Autodesk Inventor part; units mm, degrees
(part 2 of 3)
sketch "Эскиз4" plane through (0, 2, 0) normal (0, 1, 0) x (1, 0, 0)
  arc A0 (37.7453, 90.4395) -> (18.0526, 96.3229) centre (0, 0) ccw projected
  arc A1 (38.3892, 87.1795) -> (37.7453, 90.4395) centre (36.975, 88.5938) ccw projected
  line L0 (38.3892, 87.1795) -> (34.2947, 83.085) projected
  arc A2 (34.2947, 83.085) -> (34.2947, 76.014) centre (37.8302, 79.5495) ccw projected
  line L1 (34.2947, 76.014) -> (42.4264, 67.8823) projected
  line L2 (42.4264, 67.8823) -> (21.6698, 47.1257) projected
  arc A3 (21.6698, 47.1257) -> (17.9282, 43.384) centre (21.9203, 43.1335) ccw projected
  line L3 (17.9282, 43.384) -> (1.4142, 26.8701) projected
  arc A4 (-1.4142, 26.8701) -> (1.4142, 26.8701) centre (0, 28.2843) ccw projected
  line L4 (-1.4142, 26.8701) -> (-17.9282, 43.384) projected
  arc A5 (-17.9282, 43.384) -> (-21.6698, 47.1257) centre (-21.9203, 43.1335) ccw projected
  line L5 (-21.6698, 47.1257) -> (-42.4264, 67.8823) projected
  line L6 (-42.4264, 67.8823) -> (-34.2947, 76.014) projected
  arc A6 (-34.2947, 76.014) -> (-34.2947, 83.085) centre (-37.8302, 79.5495) ccw projected
  line L7 (-34.2947, 83.085) -> (-38.3892, 87.1795) projected
  arc A7 (-37.7453, 90.4395) -> (-38.3892, 87.1795) centre (-36.975, 88.5938) ccw projected
  arc A8 (-18.0526, 96.3229) -> (-37.7453, 90.4395) centre (0, 0) ccw projected
  arc A9 (-14.5, 93.3742) -> (-18.0526, 96.3229) centre (-17.5, 93.3742) ccw projected
  line L8 (-14.5, 93.3742) -> (-14.5, 87) projected
  arc A10 (-14.5, 87) -> (-11.5, 84) centre (-11.5, 87) ccw projected
  line L9 (-11.5, 84) -> (11.5, 84) projected
  arc A11 (11.5, 84) -> (14.5, 87) centre (11.5, 87) ccw projected
  line L10 (14.5, 87) -> (14.5, 93.3742) projected
  arc A12 (18.0526, 96.3229) -> (14.5, 93.3742) centre (17.5, 93.3742) ccw projected
  line L11 (8.5, 101.3496) -> (8.5, 90.5) projected
  arc A13 (7, 89) -> (8.5, 90.5) centre (7, 90.5) ccw projected
  line L12 (7, 89) -> (-7, 89) projected
  arc A14 (-8.5, 90.5) -> (-7, 89) centre (-7, 90.5) ccw projected
  line L13 (-8.5, 90.5) -> (-8.5, 101.3496) projected
  arc A15 (-8.5, 101.3496) -> (-11.8382, 104.3305) centre (-11.5, 101.3496) ccw projected
  arc A16 (-11.8382, 104.3305) -> (-48.6481, 93.0503) centre (0, 0) ccw projected
  arc A17 (-48.6481, 93.0503) -> (-49.3795, 88.2704) centre (-47.2582, 90.3917) ccw projected
  line L14 (-49.3795, 88.2704) -> (-46.3155, 85.2064) projected
  arc A18 (-46.3155, 73.8927) -> (-46.3155, 85.2064) centre (-51.9723, 79.5495) ccw projected
  line L15 (-46.3155, 73.8927) -> (-73.8927, 46.3155) projected
  arc A19 (-85.2064, 46.3155) -> (-73.8927, 46.3155) centre (-79.5495, 51.9723) ccw projected
  line L16 (-85.2064, 46.3155) -> (-88.2704, 49.3795) projected
  arc A20 (-88.2704, 49.3795) -> (-93.0503, 48.6481) centre (-90.3917, 47.2582) ccw projected
  arc A21 (-93.0503, 48.6481) -> (-93.0503, -48.6481) centre (0, 0) ccw projected
  arc A22 (-93.0503, -48.6481) -> (-88.2704, -49.3795) centre (-90.3917, -47.2582) ccw projected
  line L17 (-88.2704, -49.3795) -> (-85.2064, -46.3155) projected
  arc A23 (-73.8927, -46.3155) -> (-85.2064, -46.3155) centre (-79.5495, -51.9723) ccw projected
  line L18 (-73.8927, -46.3155) -> (-46.3155, -73.8927) projected
  arc A24 (-46.3155, -85.2064) -> (-46.3155, -73.8927) centre (-51.9723, -79.5495) ccw projected
  line L19 (-46.3155, -85.2064) -> (-49.3795, -88.2704) projected
  arc A25 (-49.3795, -88.2704) -> (-48.6481, -93.0503) centre (-47.2582, -90.3917) ccw projected
  arc A26 (-48.6481, -93.0503) -> (-45.42, -94.668) centre (0, 0) ccw projected
  arc A27 (-45.42, -94.668) -> (-43.0355, -94.1655) centre (-44.5548, -92.8648) ccw projected
  line L20 (-43.0355, -94.1655) -> (-18.3802, -65.3664) projected
  arc A28 (-17.477, -64.7643) -> (-18.3802, -65.3664) centre (-16.8609, -66.6671) ccw projected
  line L21 (-17.477, -64.7643) -> (-0.6161, -59.3045) projected
  arc A29 (0.6161, -59.3045) -> (-0.6161, -59.3045) centre (0, -61.2072) ccw projected
  line L22 (0.6161, -59.3045) -> (17.477, -64.7643) projected
  arc A30 (18.3802, -65.3664) -> (17.477, -64.7643) centre (16.8609, -66.6671) ccw projected
  line L23 (18.3802, -65.3664) -> (43.0355, -94.1655) projected
  arc A31 (43.0355, -94.1655) -> (45.42, -94.668) centre (44.5548, -92.8648) ccw projected
  arc A32 (45.42, -94.668) -> (48.6481, -93.0503) centre (0, 0) ccw projected
  arc A33 (48.6481, -93.0503) -> (49.3795, -88.2704) centre (47.2582, -90.3917) ccw projected
  line L24 (49.3795, -88.2704) -> (46.3155, -85.2064) projected
  arc A34 (46.3155, -73.8927) -> (46.3155, -85.2064) centre (51.9723, -79.5495) ccw projected
  line L25 (46.3155, -73.8927) -> (73.8927, -46.3155) projected
  arc A35 (85.2064, -46.3155) -> (73.8927, -46.3155) centre (79.5495, -51.9723) ccw projected
  line L26 (85.2064, -46.3155) -> (88.2704, -49.3795) projected
  arc A36 (88.2704, -49.3795) -> (93.0503, -48.6481) centre (90.3917, -47.2582) ccw projected
  arc A37 (93.0503, -48.6481) -> (93.0503, 48.6481) centre (0, 0) ccw projected
  arc A38 (93.0503, 48.6481) -> (88.2704, 49.3795) centre (90.3917, 47.2582) ccw projected
  line L27 (88.2704, 49.3795) -> (85.2064, 46.3155) projected
  arc A39 (73.8927, 46.3155) -> (85.2064, 46.3155) centre (79.5495, 51.9723) ccw projected
  line L28 (73.8927, 46.3155) -> (46.3155, 73.8927) projected
  arc A40 (46.3155, 85.2064) -> (46.3155, 73.8927) centre (51.9723, 79.5495) ccw projected
  line L29 (46.3155, 85.2064) -> (49.3795, 88.2704) projected
  arc A41 (49.3795, 88.2704) -> (48.6481, 93.0503) centre (47.2582, 90.3917) ccw projected
  arc A42 (48.6481, 93.0503) -> (11.8382, 104.3305) centre (0, 0) ccw projected
  arc A43 (11.8382, 104.3305) -> (8.5, 101.3496) centre (11.5, 101.3496) ccw projected
  line L30 (67.8823, -42.4264) -> (47.1257, -21.6698) projected
  arc A44 (47.1257, -21.6698) -> (43.384, -17.9282) centre (43.1335, -21.9203) ccw projected
  line L31 (43.384, -17.9282) -> (26.8701, -1.4142) projected
  arc A45 (26.8701, 1.4142) -> (26.8701, -1.4142) centre (28.2843, 0) ccw projected
  line L32 (26.8701, 1.4142) -> (43.384, 17.9282) projected
  arc A46 (43.384, 17.9282) -> (47.1257, 21.6698) centre (43.1335, 21.9203) ccw projected
  line L33 (47.1257, 21.6698) -> (67.8823, 42.4264) projected
  line L34 (67.8823, 42.4264) -> (76.014, 34.2947) projected
  arc A47 (76.014, 34.2947) -> (83.085, 34.2947) centre (79.5495, 37.8302) ccw projected
  line L35 (83.085, 34.2947) -> (87.1795, 38.3892) projected
  arc A48 (90.4395, 37.7453) -> (87.1795, 38.3892) centre (88.5938, 36.975) ccw projected
  arc A49 (90.4395, -37.7453) -> (90.4395, 37.7453) centre (0, 0) ccw projected
  arc A50 (87.1795, -38.3892) -> (90.4395, -37.7453) centre (88.5938, -36.975) ccw projected
  line L36 (87.1795, -38.3892) -> (83.085, -34.2947) projected
  arc A51 (83.085, -34.2947) -> (76.014, -34.2947) centre (79.5495, -37.8302) ccw projected
  line L37 (76.014, -34.2947) -> (67.8823, -42.4264) projected
  circle A52 centre (-37.8302, -79.5495) radius 1.6 projected
  circle A53 centre (37.8302, -79.5495) radius 1.6 projected
  circle A54 centre (20.5578, -60.8546) radius 1.55 projected
  circle A55 centre (-20.5578, -60.8546) radius 1.55 projected
  circle A56 centre (79.5495, 37.8302) radius 1.6 projected
  circle A57 centre (37.8302, 79.5495) radius 1.6 projected
  circle A58 centre (79.5495, -37.8302) radius 1.6 projected
  circle A59 centre (-79.5495, -37.8302) radius 1.6 projected
  circle A60 centre (-79.5495, 37.8302) radius 1.6 projected
  circle A61 centre (-37.8302, 79.5495) radius 1.6 projected
  circle A62 centre (22, 0) radius 1.6 projected
  circle A63 centre (0, -22) radius 1.6 projected
  circle A64 centre (-22, 0) radius 1.6 projected
  circle A65 centre (0, 22) radius 1.6 projected
  circle A66 centre (43.1335, -21.9203) radius 1.6 projected
  circle A67 centre (0, 0) radius 18 projected
  circle A68 centre (-43.1335, 21.9203) radius 1.6 projected
  circle A69 centre (-21.9203, -43.1335) radius 1.6 projected
  circle A70 centre (21.9203, 43.1335) radius 1.6 projected
  circle A71 centre (43.1335, 21.9203) radius 1.6 projected
  circle A72 centre (-43.1335, -21.9203) radius 1.6 projected
  arc A73 (-21.4111, -8.4003) -> (-8.4003, -21.4111) centre (0, 0) ccw projected
  arc A74 (-7.7166, -24.6871) -> (-8.4003, -21.4111) centre (-9.1308, -23.2729) ccw projected
  line L38 (-7.7166, -24.6871) -> (-20.8597, -37.8302) projected
  arc A75 (-23.6881, -37.8302) -> (-20.8597, -37.8302) centre (-22.2739, -36.416) ccw projected
  line L39 (-23.6881, -37.8302) -> (-37.8302, -23.6881) projected
  arc A76 (-37.8302, -20.8597) -> (-37.8302, -23.6881) centre (-36.416, -22.2739) ccw projected
  line L40 (-37.8302, -20.8597) -> (-24.6871, -7.7166) projected
  arc A77 (-21.4111, -8.4003) -> (-24.6871, -7.7166) centre (-23.2729, -9.1308) ccw projected
  circle A78 centre (21.9203, -43.1335) radius 1.6 projected
  line L41 (37.8302, 20.8597) -> (24.6871, 7.7166) projected
  arc A79 (21.4111, 8.4003) -> (24.6871, 7.7166) centre (23.2729, 9.1308) ccw projected
  arc A80 (21.4111, 8.4003) -> (8.4003, 21.4111) centre (0, 0) ccw projected
  arc A81 (7.7166, 24.6871) -> (8.4003, 21.4111) centre (9.1308, 23.2729) ccw projected
  line L42 (7.7166, 24.6871) -> (20.8597, 37.8302) projected
  arc A82 (23.6881, 37.8302) -> (20.8597, 37.8302) centre (22.2739, 36.416) ccw projected
  line L43 (23.6881, 37.8302) -> (37.8302, 23.6881) projected
  arc A83 (37.8302, 20.8597) -> (37.8302, 23.6881) centre (36.416, 22.2739) ccw projected
  arc A84 (-24.6871, 7.7166) -> (-21.4111, 8.4003) centre (-23.2729, 9.1308) ccw projected
  line L44 (-24.6871, 7.7166) -> (-37.8302, 20.8597) projected
  arc A85 (-37.8302, 23.6881) -> (-37.8302, 20.8597) centre (-36.416, 22.2739) ccw projected
  line L45 (-37.8302, 23.6881) -> (-23.6881, 37.8302) projected
  arc A86 (-20.8597, 37.8302) -> (-23.6881, 37.8302) centre (-22.2739, 36.416) ccw projected
  line L46 (-20.8597, 37.8302) -> (-7.7166, 24.6871) projected
  arc A87 (-8.4003, 21.4111) -> (-7.7166, 24.6871) centre (-9.1308, 23.2729) ccw projected
  arc A88 (-8.4003, 21.4111) -> (-21.4111, 8.4003) centre (0, 0) ccw projected
  circle A89 centre (-21.9203, 43.1335) radius 1.6 projected
  arc A90 (24.6871, -7.7166) -> (21.4111, -8.4003) centre (23.2729, -9.1308) ccw projected
  line L47 (24.6871, -7.7166) -> (37.8302, -20.8597) projected
  arc A91 (37.8302, -23.6881) -> (37.8302, -20.8597) centre (36.416, -22.2739) ccw projected
  line L48 (37.8302, -23.6881) -> (23.6881, -37.8302) projected
  arc A92 (20.8597, -37.8302) -> (23.6881, -37.8302) centre (22.2739, -36.416) ccw projected
  line L49 (20.8597, -37.8302) -> (7.7166, -24.6871) projected
  arc A93 (8.4003, -21.4111) -> (7.7166, -24.6871) centre (9.1308, -23.2729) ccw projected
  arc A94 (8.4003, -21.4111) -> (21.4111, -8.4003) centre (0, 0) ccw projected
  line L50 (46.669, -63.6396) -> (27.2236, -44.1942) projected
  arc A95 (27.2236, -41.3657) -> (27.2236, -44.1942) centre (28.6378, -42.78) ccw projected
  line L51 (27.2236, -41.3657) -> (41.3657, -27.2236) projected
  arc A96 (44.1942, -27.2236) -> (41.3657, -27.2236) centre (42.78, -28.6378) ccw projected
  line L52 (44.1942, -27.2236) -> (63.6396, -46.669) projected
  line L53 (63.6396, -46.669) -> (46.669, -63.6396) projected
  line L54 (-42.4264, -67.8823) -> (-21.6698, -47.1257) projected
  arc A97 (-21.6698, -47.1257) -> (-17.9282, -43.384) centre (-21.9203, -43.1335) ccw projected
  line L55 (-17.9282, -43.384) -> (-1.4142, -26.8701) projected
  arc A98 (1.4142, -26.8701) -> (-1.4142, -26.8701) centre (0, -28.2843) ccw projected
  line L56 (1.4142, -26.8701) -> (17.9282, -43.384) projected
  arc A99 (17.9282, -43.384) -> (21.6698, -47.1257) centre (21.9203, -43.1335) ccw projected
  line L57 (21.6698, -47.1257) -> (42.4264, -67.8823) projected
  line L58 (42.4264, -67.8823) -> (37.1244, -73.1843) projected
  arc A100 (34.1909, -73.0707) -> (37.1244, -73.1843) centre (35.7102, -71.7701) ccw projected
  line L59 (34.1909, -73.0707) -> (25.4187, -62.8242) projected
  arc A101 (24.842, -61.8893) -> (25.4187, -62.8242) centre (28.1154, -60.5155) ccw projected
  line L60 (24.842, -61.8893) -> (23.8313, -59.4808) projected
  arc A102 (23.8313, -59.4808) -> (21.0049, -57.3328) centre (20.5578, -60.8546) ccw projected
  line L61 (21.0049, -57.3328) -> (15.1585, -56.5907) projected
  arc A103 (14.5119, -56.4463) -> (15.1585, -56.5907) centre (15.6055, -53.069) ccw projected
  line L62 (14.5119, -56.4463) -> (0.6161, -51.9466) projected
  arc A104 (0.6161, -51.9466) -> (-0.6161, -51.9466) centre (0, -53.8493) ccw projected
  line L63 (-0.6161, -51.9466) -> (-14.5119, -56.4463) projected
  arc A105 (-15.1585, -56.5907) -> (-14.5119, -56.4463) centre (-15.6055, -53.069) ccw projected
  line L64 (-15.1585, -56.5907) -> (-21.0049, -57.3328) projected
  arc A106 (-21.0049, -57.3328) -> (-23.8313, -59.4808) centre (-20.5578, -60.8546) ccw projected
  line L65 (-23.8313, -59.4808) -> (-24.842, -61.8893) projected
  arc A107 (-25.4187, -62.8242) -> (-24.842, -61.8893) centre (-28.1154, -60.5155) ccw projected
  line L66 (-25.4187, -62.8242) -> (-34.1909, -73.0707) projected
  arc A108 (-37.1244, -73.1843) -> (-34.1909, -73.0707) centre (-35.7102, -71.7701) ccw projected
  line L67 (-37.1244, -73.1843) -> (-42.4264, -67.8823) projected
  line L68 (-63.6396, -46.669) -> (-44.1942, -27.2236) projected
  arc A109 (-41.3657, -27.2236) -> (-44.1942, -27.2236) centre (-42.78, -28.6378) ccw projected
  line L69 (-41.3657, -27.2236) -> (-27.2236, -41.3657) projected
  arc A110 (-27.2236, -44.1942) -> (-27.2236, -41.3657) centre (-28.6378, -42.78) ccw projected
  line L70 (-27.2236, -44.1942) -> (-46.669, -63.6396) projected
  line L71 (-46.669, -63.6396) -> (-63.6396, -46.669) projected
  line L72 (-67.8823, 42.4264) -> (-47.1257, 21.6698) projected
  arc A111 (-47.1257, 21.6698) -> (-43.384, 17.9282) centre (-43.1335, 21.9203) ccw projected
  line L73 (-43.384, 17.9282) -> (-26.8701, 1.4142) projected
  arc A112 (-26.8701, -1.4142) -> (-26.8701, 1.4142) centre (-28.2843, 0) ccw projected
  line L74 (-26.8701, -1.4142) -> (-43.384, -17.9282) projected
  arc A113 (-43.384, -17.9282) -> (-47.1257, -21.6698) centre (-43.1335, -21.9203) ccw projected
  line L75 (-47.1257, -21.6698) -> (-67.8823, -42.4264) projected
  line L76 (-67.8823, -42.4264) -> (-76.014, -34.2947) projected
  arc A114 (-76.014, -34.2947) -> (-83.085, -34.2947) centre (-79.5495, -37.8302) ccw projected
  line L77 (-83.085, -34.2947) -> (-87.1795, -38.3892) projected
  arc A115 (-90.4395, -37.7453) -> (-87.1795, -38.3892) centre (-88.5938, -36.975) ccw projected
  arc A116 (-90.4395, 37.7453) -> (-90.4395, -37.7453) centre (0, 0) ccw projected
  arc A117 (-87.1795, 38.3892) -> (-90.4395, 37.7453) centre (-88.5938, 36.975) ccw projected
  line L78 (-87.1795, 38.3892) -> (-83.085, 34.2947) projected
  arc A118 (-83.085, 34.2947) -> (-76.014, 34.2947) centre (-79.5495, 37.8302) ccw projected
  line L79 (-76.014, 34.2947) -> (-67.8823, 42.4264) projected
  line L80 (-46.669, 63.6396) -> (-27.2236, 44.1942) projected
  arc A119 (-27.2236, 41.3657) -> (-27.2236, 44.1942) centre (-28.6378, 42.78) ccw projected
  line L81 (-27.2236, 41.3657) -> (-41.3657, 27.2236) projected
  arc A120 (-44.1942, 27.2236) -> (-41.3657, 27.2236) centre (-42.78, 28.6378) ccw projected
  line L82 (-44.1942, 27.2236) -> (-63.6396, 46.669) projected
  line L83 (-63.6396, 46.669) -> (-46.669, 63.6396) projected
  line L84 (46.669, 63.6396) -> (63.6396, 46.669) projected
  line L85 (63.6396, 46.669) -> (44.1942, 27.2236) projected
  arc A121 (41.3657, 27.2236) -> (44.1942, 27.2236) centre (42.78, 28.6378) ccw projected
  line L86 (41.3657, 27.2236) -> (27.2236, 41.3657) projected
  arc A122 (27.2236, 44.1942) -> (27.2236, 41.3657) centre (28.6378, 42.78) ccw projected
  line L87 (27.2236, 44.1942) -> (46.669, 63.6396) projected
  circle A123 centre (-20.5578, -60.8546) radius 1.55 construction
  line L88 (-20.5578, -60.8546) -> (-27.9783, -53.4341) construction
  line L89 (-42.4264, -67.8823) -> (-21.6698, -47.1257) construction
  line L90 (-26.2105, -51.6664) -> (-20.5723, -57.3046)
  line L91 (-24.3148, -60.6331) -> (-29.746, -55.2019)
  line L92 (0, 0) -> (0, -61.2072) construction
  line L93 (26.2105, -51.6664) -> (20.5723, -57.3046)
  line L94 (24.3148, -60.6331) -> (29.746, -55.2019)
  point P0 (20.596, -57.2809)
  point P1 (-20.596, -57.2809)
  dimension "d100" = 5
  constraints: 12 end point, 4 point on line, 4 symmetric about line, 1 parallel, 1 perpendicular, 1 point on circle, 1 vertical, 1 other
  measures "d100" distance between parallel lines of L91 L90
extrude "Выдавливание5" add sketch "Эскиз4" against normal blind 2 contours L54 L90 L64 A106 L65 L91 | L57 L94 L60 A102 L61 L93
sketch "Эскиз5" plane through (0, 2, 0) normal (0, 1, 0) x (1, 0, 0)
  line L0 (29.746, -55.2019) -> (42.4264, -67.8823) construction
  line L1 (42.4264, -67.8823) -> (37.1244, -73.1843) construction
  arc A0 (34.1909, -73.0707) -> (37.1244, -73.1843) centre (35.7102, -71.7701) ccw construction
  line L2 (34.1909, -73.0707) -> (25.4187, -62.8242) construction
  arc A1 (24.842, -61.8893) -> (25.4187, -62.8242) centre (28.1154, -60.5155) ccw construction
  line L3 (24.842, -61.8893) -> (24.3148, -60.6331) construction
  line L4 (24.3148, -60.6331) -> (29.746, -55.2019) construction
  line L5 (26.2105, -51.6664) -> (20.596, -57.2809) construction
  line L6 (20.596, -57.2809) -> (15.1585, -56.5907) construction
  arc A2 (14.5119, -56.4463) -> (15.1585, -56.5907) centre (15.6055, -53.069) ccw construction
  line L7 (14.5119, -56.4463) -> (0.6161, -51.9466) construction
  arc A3 (0.6161, -51.9466) -> (-0.6161, -51.9466) centre (0, -53.8493) ccw construction
  line L8 (-0.6161, -51.9466) -> (-14.5119, -56.4463) construction
  arc A4 (-15.1585, -56.5907) -> (-14.5119, -56.4463) centre (-15.6055, -53.069) ccw construction
  line L9 (-15.1585, -56.5907) -> (-20.596, -57.2809) construction
  line L10 (-20.596, -57.2809) -> (-26.2105, -51.6664) construction
  line L11 (-26.2105, -51.6664) -> (-21.6698, -47.1257) construction
  arc A5 (-21.6698, -47.1257) -> (-17.9282, -43.384) centre (-21.9203, -43.1335) ccw construction
  line L12 (-17.9282, -43.384) -> (-1.4142, -26.8701) construction
  arc A6 (1.4142, -26.8701) -> (-1.4142, -26.8701) centre (0, -28.2843) ccw construction
  line L13 (1.4142, -26.8701) -> (17.9282, -43.384) construction
  arc A7 (17.9282, -43.384) -> (21.6698, -47.1257) centre (21.9203, -43.1335) ccw construction
  line L14 (21.6698, -47.1257) -> (26.2105, -51.6664) construction
  arc A8 (37.7453, 90.4395) -> (18.0526, 96.3229) centre (0, 0) ccw construction
  arc A9 (38.3892, 87.1795) -> (37.7453, 90.4395) centre (36.975, 88.5938) ccw construction
  line L15 (38.3892, 87.1795) -> (34.2947, 83.085) construction
  arc A10 (34.2947, 83.085) -> (34.2947, 76.014) centre (37.8302, 79.5495) ccw construction
  line L16 (34.2947, 76.014) -> (42.4264, 67.8823) construction
  line L17 (42.4264, 67.8823) -> (21.6698, 47.1257) construction
  arc A11 (21.6698, 47.1257) -> (17.9282, 43.384) centre (21.9203, 43.1335) ccw construction
  line L18 (17.9282, 43.384) -> (1.4142, 26.8701) construction
  arc A12 (-1.4142, 26.8701) -> (1.4142, 26.8701) centre (0, 28.2843) ccw construction
  line L19 (-1.4142, 26.8701) -> (-17.9282, 43.384) construction
  arc A13 (-17.9282, 43.384) -> (-21.6698, 47.1257) centre (-21.9203, 43.1335) ccw construction
  line L20 (-21.6698, 47.1257) -> (-42.4264, 67.8823) construction
  line L21 (-42.4264, 67.8823) -> (-34.2947, 76.014) construction
  arc A14 (-34.2947, 76.014) -> (-34.2947, 83.085) centre (-37.8302, 79.5495) ccw construction
  line L22 (-34.2947, 83.085) -> (-38.3892, 87.1795) construction
  arc A15 (-37.7453, 90.4395) -> (-38.3892, 87.1795) centre (-36.975, 88.5938) ccw construction
  arc A16 (-18.0526, 96.3229) -> (-37.7453, 90.4395) centre (0, 0) ccw construction
  arc A17 (-14.5, 93.3742) -> (-18.0526, 96.3229) centre (-17.5, 93.3742) ccw construction
  line L23 (-14.5, 93.3742) -> (-14.5, 87) construction
  arc A18 (-14.5, 87) -> (-11.5, 84) centre (-11.5, 87) ccw construction
  line L24 (-11.5, 84) -> (11.5, 84) construction
  arc A19 (11.5, 84) -> (14.5, 87) centre (11.5, 87) ccw construction
  line L25 (14.5, 87) -> (14.5, 93.3742) construction
  arc A20 (18.0526, 96.3229) -> (14.5, 93.3742) centre (17.5, 93.3742) ccw construction
  line L26 (8.5, 101.3496) -> (8.5, 90.5) construction
  arc A21 (7, 89) -> (8.5, 90.5) centre (7, 90.5) ccw construction
  line L27 (7, 89) -> (-7, 89) construction
  arc A22 (-8.5, 90.5) -> (-7, 89) centre (-7, 90.5) ccw construction
  line L28 (-8.5, 90.5) -> (-8.5, 101.3496) construction
  arc A23 (-8.5, 101.3496) -> (-11.8382, 104.3305) centre (-11.5, 101.3496) ccw construction
  arc A24 (-11.8382, 104.3305) -> (-48.6481, 93.0503) centre (0, 0) ccw construction
  arc A25 (-48.6481, 93.0503) -> (-49.3795, 88.2704) centre (-47.2582, 90.3917) ccw construction
  line L29 (-49.3795, 88.2704) -> (-46.3155, 85.2064) construction
  arc A26 (-46.3155, 73.8927) -> (-46.3155, 85.2064) centre (-51.9723, 79.5495) ccw construction
  line L30 (-46.3155, 73.8927) -> (-73.8927, 46.3155) construction
  arc A27 (-85.2064, 46.3155) -> (-73.8927, 46.3155) centre (-79.5495, 51.9723) ccw construction
  line L31 (-85.2064, 46.3155) -> (-88.2704, 49.3795) construction
  arc A28 (-88.2704, 49.3795) -> (-93.0503, 48.6481) centre (-90.3917, 47.2582) ccw construction
  arc A29 (-93.0503, 48.6481) -> (-93.0503, -48.6481) centre (0, 0) ccw construction
  arc A30 (-93.0503, -48.6481) -> (-88.2704, -49.3795) centre (-90.3917, -47.2582) ccw construction
  line L32 (-88.2704, -49.3795) -> (-85.2064, -46.3155) construction
  arc A31 (-73.8927, -46.3155) -> (-85.2064, -46.3155) centre (-79.5495, -51.9723) ccw construction
  line L33 (-73.8927, -46.3155) -> (-46.3155, -73.8927) construction
  arc A32 (-46.3155, -85.2064) -> (-46.3155, -73.8927) centre (-51.9723, -79.5495) ccw construction
  line L34 (-46.3155, -85.2064) -> (-49.3795, -88.2704) construction
  arc A33 (-49.3795, -88.2704) -> (-48.6481, -93.0503) centre (-47.2582, -90.3917) ccw construction
  arc A34 (-48.6481, -93.0503) -> (-45.42, -94.668) centre (0, 0) ccw construction
  arc A35 (-45.42, -94.668) -> (-43.0355, -94.1655) centre (-44.5548, -92.8648) ccw construction
  line L35 (-43.0355, -94.1655) -> (-18.3802, -65.3664) construction
  arc A36 (-17.477, -64.7643) -> (-18.3802, -65.3664) centre (-16.8609, -66.6671) ccw construction
  line L36 (-17.477, -64.7643) -> (-0.6161, -59.3045) construction
  arc A37 (0.6161, -59.3045) -> (-0.6161, -59.3045) centre (0, -61.2072) ccw construction
  line L37 (0.6161, -59.3045) -> (17.477, -64.7643) construction
  arc A38 (18.3802, -65.3664) -> (17.477, -64.7643) centre (16.8609, -66.6671) ccw construction
  line L38 (18.3802, -65.3664) -> (43.0355, -94.1655) construction
  arc A39 (43.0355, -94.1655) -> (45.42, -94.668) centre (44.5548, -92.8648) ccw construction
  arc A40 (45.42, -94.668) -> (48.6481, -93.0503) centre (0, 0) ccw construction
  arc A41 (48.6481, -93.0503) -> (49.3795, -88.2704) centre (47.2582, -90.3917) ccw construction
  line L39 (49.3795, -88.2704) -> (46.3155, -85.2064) construction
  arc A42 (46.3155, -73.8927) -> (46.3155, -85.2064) centre (51.9723, -79.5495) ccw construction
  line L40 (46.3155, -73.8927) -> (73.8927, -46.3155) construction
  arc A43 (85.2064, -46.3155) -> (73.8927, -46.3155) centre (79.5495, -51.9723) ccw construction
  line L41 (85.2064, -46.3155) -> (88.2704, -49.3795) construction
  arc A44 (88.2704, -49.3795) -> (93.0503, -48.6481) centre (90.3917, -47.2582) ccw construction
  arc A45 (93.0503, -48.6481) -> (93.0503, 48.6481) centre (0, 0) ccw construction
  arc A46 (93.0503, 48.6481) -> (88.2704, 49.3795) centre (90.3917, 47.2582) ccw construction
  line L42 (88.2704, 49.3795) -> (85.2064, 46.3155) construction
  arc A47 (73.8927, 46.3155) -> (85.2064, 46.3155) centre (79.5495, 51.9723) ccw construction
  line L43 (73.8927, 46.3155) -> (46.3155, 73.8927) construction
  arc A48 (46.3155, 85.2064) -> (46.3155, 73.8927) centre (51.9723, 79.5495) ccw construction
  line L44 (46.3155, 85.2064) -> (49.3795, 88.2704) construction
  arc A49 (49.3795, 88.2704) -> (48.6481, 93.0503) centre (47.2582, 90.3917) ccw construction
  arc A50 (48.6481, 93.0503) -> (11.8382, 104.3305) centre (0, 0) ccw construction
  arc A51 (11.8382, 104.3305) -> (8.5, 101.3496) centre (11.5, 101.3496) ccw construction
  line L45 (67.8823, -42.4264) -> (47.1257, -21.6698) construction
  arc A52 (47.1257, -21.6698) -> (43.384, -17.9282) centre (43.1335, -21.9203) ccw construction
  line L46 (43.384, -17.9282) -> (26.8701, -1.4142) construction
  arc A53 (26.8701, 1.4142) -> (26.8701, -1.4142) centre (28.2843, 0) ccw construction
  line L47 (26.8701, 1.4142) -> (43.384, 17.9282) construction
  arc A54 (43.384, 17.9282) -> (47.1257, 21.6698) centre (43.1335, 21.9203) ccw construction
  line L48 (47.1257, 21.6698) -> (67.8823, 42.4264) construction
  line L49 (67.8823, 42.4264) -> (76.014, 34.2947) construction
  arc A55 (76.014, 34.2947) -> (83.085, 34.2947) centre (79.5495, 37.8302) ccw construction
  line L50 (83.085, 34.2947) -> (87.1795, 38.3892) construction
  arc A56 (90.4395, 37.7453) -> (87.1795, 38.3892) centre (88.5938, 36.975) ccw construction
  arc A57 (90.4395, -37.7453) -> (90.4395, 37.7453) centre (0, 0) ccw construction
  arc A58 (87.1795, -38.3892) -> (90.4395, -37.7453) centre (88.5938, -36.975) ccw construction
  line L51 (87.1795, -38.3892) -> (83.085, -34.2947) construction
  arc A59 (83.085, -34.2947) -> (76.014, -34.2947) centre (79.5495, -37.8302) ccw construction
  line L52 (76.014, -34.2947) -> (67.8823, -42.4264) construction
  circle A60 centre (-37.8302, -79.5495) radius 1.6 construction
  circle A61 centre (37.8302, -79.5495) radius 1.6 construction
  circle A62 centre (20.5578, -60.8546) radius 1.55 construction
  circle A63 centre (-20.5578, -60.8546) radius 1.55 construction
  circle A64 centre (79.5495, 37.8302) radius 1.6 construction
  circle A65 centre (37.8302, 79.5495) radius 1.6 construction
  circle A66 centre (79.5495, -37.8302) radius 1.6 construction
  circle A67 centre (-79.5495, -37.8302) radius 1.6 construction
  circle A68 centre (-79.5495, 37.8302) radius 1.6 construction
  circle A69 centre (-37.8302, 79.5495) radius 1.6 construction
  circle A70 centre (22, 0) radius 1.6 construction
  circle A71 centre (0, -22) radius 1.6 construction
  circle A72 centre (-22, 0) radius 1.6 construction
  circle A73 centre (0, 22) radius 1.6 construction
  circle A74 centre (43.1335, -21.9203) radius 1.6 construction
  circle A75 centre (0, 0) radius 18 construction
  circle A76 centre (-43.1335, 21.9203) radius 1.6 construction
  circle A77 centre (-21.9203, -43.1335) radius 1.6 construction
  circle A78 centre (21.9203, 43.1335) radius 1.6 construction
  circle A79 centre (43.1335, 21.9203) radius 1.6 construction
  circle A80 centre (-43.1335, -21.9203) radius 1.6 construction
  arc A81 (-21.4111, -8.4003) -> (-8.4003, -21.4111) centre (0, 0) ccw construction
  arc A82 (-7.7166, -24.6871) -> (-8.4003, -21.4111) centre (-9.1308, -23.2729) ccw construction
  line L53 (-7.7166, -24.6871) -> (-20.8597, -37.8302) construction
  arc A83 (-23.6881, -37.8302) -> (-20.8597, -37.8302) centre (-22.2739, -36.416) ccw construction
  line L54 (-23.6881, -37.8302) -> (-37.8302, -23.6881) construction
  arc A84 (-37.8302, -20.8597) -> (-37.8302, -23.6881) centre (-36.416, -22.2739) ccw construction
  line L55 (-37.8302, -20.8597) -> (-24.6871, -7.7166) construction
  arc A85 (-21.4111, -8.4003) -> (-24.6871, -7.7166) centre (-23.2729, -9.1308) ccw construction
  circle A86 centre (21.9203, -43.1335) radius 1.6 construction
  line L56 (37.8302, 20.8597) -> (24.6871, 7.7166) construction
  arc A87 (21.4111, 8.4003) -> (24.6871, 7.7166) centre (23.2729, 9.1308) ccw construction
  arc A88 (21.4111, 8.4003) -> (8.4003, 21.4111) centre (0, 0) ccw construction
  arc A89 (7.7166, 24.6871) -> (8.4003, 21.4111) centre (9.1308, 23.2729) ccw construction
  line L57 (7.7166, 24.6871) -> (20.8597, 37.8302) construction
  arc A90 (23.6881, 37.8302) -> (20.8597, 37.8302) centre (22.2739, 36.416) ccw construction
  line L58 (23.6881, 37.8302) -> (37.8302, 23.6881) construction
  arc A91 (37.8302, 20.8597) -> (37.8302, 23.6881) centre (36.416, 22.2739) ccw construction
  arc A92 (-24.6871, 7.7166) -> (-21.4111, 8.4003) centre (-23.2729, 9.1308) ccw construction
  line L59 (-24.6871, 7.7166) -> (-37.8302, 20.8597) construction
  arc A93 (-37.8302, 23.6881) -> (-37.8302, 20.8597) centre (-36.416, 22.2739) ccw construction
  line L60 (-37.8302, 23.6881) -> (-23.6881, 37.8302) construction
  arc A94 (-20.8597, 37.8302) -> (-23.6881, 37.8302) centre (-22.2739, 36.416) ccw construction
  line L61 (-20.8597, 37.8302) -> (-7.7166, 24.6871) construction
  arc A95 (-8.4003, 21.4111) -> (-7.7166, 24.6871) centre (-9.1308, 23.2729) ccw construction
  arc A96 (-8.4003, 21.4111) -> (-21.4111, 8.4003) centre (0, 0) ccw construction
  circle A97 centre (-21.9203, 43.1335) radius 1.6 construction
  arc A98 (24.6871, -7.7166) -> (21.4111, -8.4003) centre (23.2729, -9.1308) ccw construction
  line L62 (24.6871, -7.7166) -> (37.8302, -20.8597) construction
  arc A99 (37.8302, -23.6881) -> (37.8302, -20.8597) centre (36.416, -22.2739) ccw construction
  line L63 (37.8302, -23.6881) -> (23.6881, -37.8302) construction
  arc A100 (20.8597, -37.8302) -> (23.6881, -37.8302) centre (22.2739, -36.416) ccw construction
  line L64 (20.8597, -37.8302) -> (7.7166, -24.6871) construction
  arc A101 (8.4003, -21.4111) -> (7.7166, -24.6871) centre (9.1308, -23.2729) ccw construction
  arc A102 (8.4003, -21.4111) -> (21.4111, -8.4003) centre (0, 0) ccw construction
  line L65 (46.669, -63.6396) -> (27.2236, -44.1942) construction
  arc A103 (27.2236, -41.3657) -> (27.2236, -44.1942) centre (28.6378, -42.78) ccw construction
  line L66 (27.2236, -41.3657) -> (41.3657, -27.2236) construction
  arc A104 (44.1942, -27.2236) -> (41.3657, -27.2236) centre (42.78, -28.6378) ccw construction
  line L67 (44.1942, -27.2236) -> (63.6396, -46.669) construction
  line L68 (63.6396, -46.669) -> (46.669, -63.6396) construction
  line L69 (-29.746, -55.2019) -> (-24.3148, -60.6331) construction
  line L70 (-24.3148, -60.6331) -> (-24.842, -61.8893) construction
  arc A105 (-25.4187, -62.8242) -> (-24.842, -61.8893) centre (-28.1154, -60.5155) ccw construction
  line L71 (-25.4187, -62.8242) -> (-34.1909, -73.0707) construction
  arc A106 (-37.1244, -73.1843) -> (-34.1909, -73.0707) centre (-35.7102, -71.7701) ccw construction
  line L72 (-37.1244, -73.1843) -> (-42.4264, -67.8823) construction
  line L73 (-42.4264, -67.8823) -> (-29.746, -55.2019) construction
  line L74 (-63.6396, -46.669) -> (-44.1942, -27.2236) construction
  arc A107 (-41.3657, -27.2236) -> (-44.1942, -27.2236) centre (-42.78, -28.6378) ccw construction
  line L75 (-41.3657, -27.2236) -> (-27.2236, -41.3657) construction
  arc A108 (-27.2236, -44.1942) -> (-27.2236, -41.3657) centre (-28.6378, -42.78) ccw construction
  line L76 (-27.2236, -44.1942) -> (-46.669, -63.6396) construction
  line L77 (-46.669, -63.6396) -> (-63.6396, -46.669) construction
  line L78 (-67.8823, 42.4264) -> (-47.1257, 21.6698) construction
  arc A109 (-47.1257, 21.6698) -> (-43.384, 17.9282) centre (-43.1335, 21.9203) ccw construction
  line L79 (-43.384, 17.9282) -> (-26.8701, 1.4142) construction
  arc A110 (-26.8701, -1.4142) -> (-26.8701, 1.4142) centre (-28.2843, 0) ccw construction
  line L80 (-26.8701, -1.4142) -> (-43.384, -17.9282) construction
  arc A111 (-43.384, -17.9282) -> (-47.1257, -21.6698) centre (-43.1335, -21.9203) ccw construction
  line L81 (-47.1257, -21.6698) -> (-67.8823, -42.4264) construction
  line L82 (-67.8823, -42.4264) -> (-76.014, -34.2947) construction
  arc A112 (-76.014, -34.2947) -> (-83.085, -34.2947) centre (-79.5495, -37.8302) ccw construction
  line L83 (-83.085, -34.2947) -> (-87.1795, -38.3892) construction
  arc A113 (-90.4395, -37.7453) -> (-87.1795, -38.3892) centre (-88.5938, -36.975) ccw construction
  arc A114 (-90.4395, 37.7453) -> (-90.4395, -37.7453) centre (0, 0) ccw construction
  arc A115 (-87.1795, 38.3892) -> (-90.4395, 37.7453) centre (-88.5938, 36.975) ccw construction
  line L84 (-87.1795, 38.3892) -> (-83.085, 34.2947) construction
  arc A116 (-83.085, 34.2947) -> (-76.014, 34.2947) centre (-79.5495, 37.8302) ccw construction
  line L85 (-76.014, 34.2947) -> (-67.8823, 42.4264) construction
  line L86 (-46.669, 63.6396) -> (-27.2236, 44.1942) construction
  arc A117 (-27.2236, 41.3657) -> (-27.2236, 44.1942) centre (-28.6378, 42.78) ccw construction
  line L87 (-27.2236, 41.3657) -> (-41.3657, 27.2236) construction
  arc A118 (-44.1942, 27.2236) -> (-41.3657, 27.2236) centre (-42.78, 28.6378) ccw construction
  line L88 (-44.1942, 27.2236) -> (-63.6396, 46.669) construction
  line L89 (-63.6396, 46.669) -> (-46.669, 63.6396) construction
  line L90 (46.669, 63.6396) -> (63.6396, 46.669) construction
  line L91 (63.6396, 46.669) -> (44.1942, 27.2236) construction
  arc A119 (41.3657, 27.2236) -> (44.1942, 27.2236) centre (42.78, 28.6378) ccw construction
  line L92 (41.3657, 27.2236) -> (27.2236, 41.3657) construction
  arc A120 (27.2236, 44.1942) -> (27.2236, 41.3657) centre (28.6378, 42.78) ccw construction
  line L93 (27.2236, 44.1942) -> (46.669, 63.6396) construction
  arc A121 (-93.0503, 48.6481) -> (-93.0503, -48.6481) centre (0, 0) ccw construction
  line L94 (-105, 0) -> (-101, 0) construction
  circle A122 centre (-101, 0) radius 4
  circle A123 centre (-101, 0) radius 1.6
  circle A124 centre (0, 0) radius 18 construction
  line L95 (0, 18) -> (0, -18) construction
  circle A125 centre (101, 0) radius 1.6
  circle A126 centre (101, 0) radius 4
  dimension "d104" = 4
  dimension "d105" = 8
  dimension "d106" = 3.2
  dimension "d109" = 101
  constraints: 4 centre point, 4 end point, 3 point on circle, 2 coincident, 2 symmetric about line, 1 horizontal, 1 vertical, 2 other
  measures "d104" distance of L94.start L94.end
  measures "d105" diameter of A122
  measures "d106" diameter of A123
  measures "d109" distance of L94.end point (0, 0)
extrude "Выдавливание7" add sketch "Эскиз5" against normal blind 2
extrude "Выдавливание8" cut sketch "Эскиз5" against normal blind 2 contours A123 | A125
sketch "Эскиз6" plane through (0, 2, 0) normal (0, 1, 0) x (1, 0, 0)
  circle A0 centre (-101, 0) radius 1.6 construction
  circle A1 centre (101, 0) radius 1.6 construction
  circle A2 centre (-101, 0) radius 1.6 construction
  arc A3 (90.4395, -37.7453) -> (97.9653, -2.6059) centre (0, 0) ccw construction
  arc A4 (87.1795, -38.3892) -> (90.4395, -37.7453) centre (88.5938, -36.975) ccw construction
  line L0 (87.1795, -38.3892) -> (83.085, -34.2947) construction
  arc A5 (83.085, -34.2947) -> (76.014, -34.2947) centre (79.5495, -37.8302) ccw construction
  line L1 (76.014, -34.2947) -> (67.8823, -42.4264) construction
  line L2 (67.8823, -42.4264) -> (47.1257, -21.6698) construction
  arc A6 (47.1257, -21.6698) -> (43.384, -17.9282) centre (43.1335, -21.9203) ccw construction
  line L3 (43.384, -17.9282) -> (26.8701, -1.4142) construction
  arc A7 (26.8701, 1.4142) -> (26.8701, -1.4142) centre (28.2843, 0) ccw construction
  line L4 (26.8701, 1.4142) -> (43.384, 17.9282) construction
  arc A8 (43.384, 17.9282) -> (47.1257, 21.6698) centre (43.1335, 21.9203) ccw construction
  line L5 (47.1257, 21.6698) -> (67.8823, 42.4264) construction
  line L6 (67.8823, 42.4264) -> (76.014, 34.2947) construction
  arc A9 (76.014, 34.2947) -> (83.085, 34.2947) centre (79.5495, 37.8302) ccw construction
  line L7 (83.085, 34.2947) -> (87.1795, 38.3892) construction
  arc A10 (90.4395, 37.7453) -> (87.1795, 38.3892) centre (88.5938, 36.975) ccw construction
  arc A11 (97.9653, 2.6059) -> (90.4395, 37.7453) centre (0, 0) ccw construction
  arc A12 (97.9653, 2.6059) -> (97.9653, -2.6059) centre (101, 0) ccw construction
  line L8 (46.669, 63.6396) -> (63.6396, 46.669) construction
  line L9 (63.6396, 46.669) -> (44.1942, 27.2236) construction
  arc A13 (41.3657, 27.2236) -> (44.1942, 27.2236) centre (42.78, 28.6378) ccw construction
  line L10 (41.3657, 27.2236) -> (27.2236, 41.3657) construction
  arc A14 (27.2236, 44.1942) -> (27.2236, 41.3657) centre (28.6378, 42.78) ccw construction
  line L11 (27.2236, 44.1942) -> (46.669, 63.6396) construction
  line L12 (-46.669, 63.6396) -> (-27.2236, 44.1942) construction
  arc A15 (-27.2236, 41.3657) -> (-27.2236, 44.1942) centre (-28.6378, 42.78) ccw construction
  line L13 (-27.2236, 41.3657) -> (-41.3657, 27.2236) construction
  arc A16 (-44.1942, 27.2236) -> (-41.3657, 27.2236) centre (-42.78, 28.6378) ccw construction
  line L14 (-44.1942, 27.2236) -> (-63.6396, 46.669) construction
  line L15 (-63.6396, 46.669) -> (-46.669, 63.6396) construction
  line L16 (-63.6396, -46.669) -> (-44.1942, -27.2236) construction
  arc A17 (-41.3657, -27.2236) -> (-44.1942, -27.2236) centre (-42.78, -28.6378) ccw construction
  line L17 (-41.3657, -27.2236) -> (-27.2236, -41.3657) construction
  arc A18 (-27.2236, -44.1942) -> (-27.2236, -41.3657) centre (-28.6378, -42.78) ccw construction
  line L18 (-27.2236, -44.1942) -> (-46.669, -63.6396) construction
  line L19 (-46.669, -63.6396) -> (-63.6396, -46.669) construction
  line L20 (-29.746, -55.2019) -> (-24.3148, -60.6331) construction
  line L21 (-24.3148, -60.6331) -> (-24.842, -61.8893) construction
  arc A19 (-25.4187, -62.8242) -> (-24.842, -61.8893) centre (-28.1154, -60.5155) ccw construction
  line L22 (-25.4187, -62.8242) -> (-34.1909, -73.0707) construction
  arc A20 (-37.1244, -73.1843) -> (-34.1909, -73.0707) centre (-35.7102, -71.7701) ccw construction
  line L23 (-37.1244, -73.1843) -> (-42.4264, -67.8823) construction
  line L24 (-42.4264, -67.8823) -> (-29.746, -55.2019) construction
  line L25 (46.669, -63.6396) -> (27.2236, -44.1942) construction
  arc A21 (27.2236, -41.3657) -> (27.2236, -44.1942) centre (28.6378, -42.78) ccw construction
  line L26 (27.2236, -41.3657) -> (41.3657, -27.2236) construction
  arc A22 (44.1942, -27.2236) -> (41.3657, -27.2236) centre (42.78, -28.6378) ccw construction
  line L27 (44.1942, -27.2236) -> (63.6396, -46.669) construction
  line L28 (63.6396, -46.669) -> (46.669, -63.6396) construction
  arc A23 (24.6871, -7.7166) -> (21.4111, -8.4003) centre (23.2729, -9.1308) ccw construction
  line L29 (24.6871, -7.7166) -> (37.8302, -20.8597) construction
  arc A24 (37.8302, -23.6881) -> (37.8302, -20.8597) centre (36.416, -22.2739) ccw construction
  line L30 (37.8302, -23.6881) -> (23.6881, -37.8302) construction
  arc A25 (20.8597, -37.8302) -> (23.6881, -37.8302) centre (22.2739, -36.416) ccw construction
  line L31 (20.8597, -37.8302) -> (7.7166, -24.6871) construction
  arc A26 (8.4003, -21.4111) -> (7.7166, -24.6871) centre (9.1308, -23.2729) ccw construction
  arc A27 (8.4003, -21.4111) -> (21.4111, -8.4003) centre (0, 0) ccw construction
  circle A28 centre (-21.9203, 43.1335) radius 1.6 construction
  arc A29 (-24.6871, 7.7166) -> (-21.4111, 8.4003) centre (-23.2729, 9.1308) ccw construction
  line L32 (-24.6871, 7.7166) -> (-37.8302, 20.8597) construction
  arc A30 (-37.8302, 23.6881) -> (-37.8302, 20.8597) centre (-36.416, 22.2739) ccw construction
  line L33 (-37.8302, 23.6881) -> (-23.6881, 37.8302) construction
  arc A31 (-20.8597, 37.8302) -> (-23.6881, 37.8302) centre (-22.2739, 36.416) ccw construction
  line L34 (-20.8597, 37.8302) -> (-7.7166, 24.6871) construction
  arc A32 (-8.4003, 21.4111) -> (-7.7166, 24.6871) centre (-9.1308, 23.2729) ccw construction
  arc A33 (-8.4003, 21.4111) -> (-21.4111, 8.4003) centre (0, 0) ccw construction
  line L35 (37.8302, 20.8597) -> (24.6871, 7.7166) construction
  arc A34 (21.4111, 8.4003) -> (24.6871, 7.7166) centre (23.2729, 9.1308) ccw construction
  arc A35 (21.4111, 8.4003) -> (8.4003, 21.4111) centre (0, 0) ccw construction
  arc A36 (7.7166, 24.6871) -> (8.4003, 21.4111) centre (9.1308, 23.2729) ccw construction
  line L36 (7.7166, 24.6871) -> (20.8597, 37.8302) construction
  arc A37 (23.6881, 37.8302) -> (20.8597, 37.8302) centre (22.2739, 36.416) ccw construction
  line L37 (23.6881, 37.8302) -> (37.8302, 23.6881) construction
  arc A38 (37.8302, 20.8597) -> (37.8302, 23.6881) centre (36.416, 22.2739) ccw construction
  circle A39 centre (21.9203, -43.1335) radius 1.6 construction
  arc A40 (-21.4111, -8.4003) -> (-8.4003, -21.4111) centre (0, 0) ccw construction
  arc A41 (-7.7166, -24.6871) -> (-8.4003, -21.4111) centre (-9.1308, -23.2729) ccw construction
  line L38 (-7.7166, -24.6871) -> (-20.8597, -37.8302) construction
  arc A42 (-23.6881, -37.8302) -> (-20.8597, -37.8302) centre (-22.2739, -36.416) ccw construction
  line L39 (-23.6881, -37.8302) -> (-37.8302, -23.6881) construction
  arc A43 (-37.8302, -20.8597) -> (-37.8302, -23.6881) centre (-36.416, -22.2739) ccw construction
  line L40 (-37.8302, -20.8597) -> (-24.6871, -7.7166) construction
  arc A44 (-21.4111, -8.4003) -> (-24.6871, -7.7166) centre (-23.2729, -9.1308) ccw construction
  circle A45 centre (-43.1335, -21.9203) radius 1.6 construction
  circle A46 centre (43.1335, 21.9203) radius 1.6 construction
  circle A47 centre (21.9203, 43.1335) radius 1.6 construction
  circle A48 centre (-21.9203, -43.1335) radius 1.6 construction
  circle A49 centre (-43.1335, 21.9203) radius 1.6 construction
  circle A50 centre (0, 0) radius 18 construction
  circle A51 centre (43.1335, -21.9203) radius 1.6 construction
  circle A52 centre (0, 22) radius 1.6 construction
  circle A53 centre (-22, 0) radius 1.6 construction
  circle A54 centre (0, -22) radius 1.6 construction
  circle A55 centre (22, 0) radius 1.6 construction
  circle A56 centre (-37.8302, 79.5495) radius 1.6 construction
  circle A57 centre (-79.5495, 37.8302) radius 1.6 construction
  circle A58 centre (-79.5495, -37.8302) radius 1.6 construction
  circle A59 centre (79.5495, -37.8302) radius 1.6 construction
  circle A60 centre (37.8302, 79.5495) radius 1.6 construction
  circle A61 centre (79.5495, 37.8302) radius 1.6 construction
  circle A62 centre (-20.5578, -60.8546) radius 1.55 construction
  circle A63 centre (20.5578, -60.8546) radius 1.55 construction
  circle A64 centre (37.8302, -79.5495) radius 1.6 construction
  circle A65 centre (-37.8302, -79.5495) radius 1.6 construction
  arc A66 (37.7453, 90.4395) -> (18.0526, 96.3229) centre (0, 0) ccw construction
  arc A67 (38.3892, 87.1795) -> (37.7453, 90.4395) centre (36.975, 88.5938) ccw construction
  line L41 (38.3892, 87.1795) -> (34.2947, 83.085) construction
  arc A68 (34.2947, 83.085) -> (34.2947, 76.014) centre (37.8302, 79.5495) ccw construction
  line L42 (34.2947, 76.014) -> (42.4264, 67.8823) construction
  line L43 (42.4264, 67.8823) -> (21.6698, 47.1257) construction
  arc A69 (21.6698, 47.1257) -> (17.9282, 43.384) centre (21.9203, 43.1335) ccw construction
  line L44 (17.9282, 43.384) -> (1.4142, 26.8701) construction
  arc A70 (-1.4142, 26.8701) -> (1.4142, 26.8701) centre (0, 28.2843) ccw construction
  line L45 (-1.4142, 26.8701) -> (-17.9282, 43.384) construction
  arc A71 (-17.9282, 43.384) -> (-21.6698, 47.1257) centre (-21.9203, 43.1335) ccw construction
  line L46 (-21.6698, 47.1257) -> (-42.4264, 67.8823) construction
  line L47 (-42.4264, 67.8823) -> (-34.2947, 76.014) construction
  arc A72 (-34.2947, 76.014) -> (-34.2947, 83.085) centre (-37.8302, 79.5495) ccw construction
  line L48 (-34.2947, 83.085) -> (-38.3892, 87.1795) construction
  arc A73 (-37.7453, 90.4395) -> (-38.3892, 87.1795) centre (-36.975, 88.5938) ccw construction
  arc A74 (-18.0526, 96.3229) -> (-37.7453, 90.4395) centre (0, 0) ccw construction
  arc A75 (-14.5, 93.3742) -> (-18.0526, 96.3229) centre (-17.5, 93.3742) ccw construction
  line L49 (-14.5, 93.3742) -> (-14.5, 87) construction
  arc A76 (-14.5, 87) -> (-11.5, 84) centre (-11.5, 87) ccw construction
  line L50 (-11.5, 84) -> (11.5, 84) construction
  arc A77 (11.5, 84) -> (14.5, 87) centre (11.5, 87) ccw construction
  line L51 (14.5, 87) -> (14.5, 93.3742) construction
  arc A78 (18.0526, 96.3229) -> (14.5, 93.3742) centre (17.5, 93.3742) ccw construction
  line L52 (26.2105, -51.6664) -> (20.596, -57.2809) construction
  line L53 (20.596, -57.2809) -> (15.1585, -56.5907) construction
  arc A79 (14.5119, -56.4463) -> (15.1585, -56.5907) centre (15.6055, -53.069) ccw construction
  line L54 (14.5119, -56.4463) -> (0.6161, -51.9466) construction
  arc A80 (0.6161, -51.9466) -> (-0.6161, -51.9466) centre (0, -53.8493) ccw construction
  line L55 (-0.6161, -51.9466) -> (-14.5119, -56.4463) construction
  arc A81 (-15.1585, -56.5907) -> (-14.5119, -56.4463) centre (-15.6055, -53.069) ccw construction
  line L56 (-15.1585, -56.5907) -> (-20.596, -57.2809) construction
  line L57 (-20.596, -57.2809) -> (-26.2105, -51.6664) construction
  line L58 (-26.2105, -51.6664) -> (-21.6698, -47.1257) construction
  arc A82 (-21.6698, -47.1257) -> (-17.9282, -43.384) centre (-21.9203, -43.1335) ccw construction
  line L59 (-17.9282, -43.384) -> (-1.4142, -26.8701) construction
  arc A83 (1.4142, -26.8701) -> (-1.4142, -26.8701) centre (0, -28.2843) ccw construction
  line L60 (1.4142, -26.8701) -> (17.9282, -43.384) construction
  arc A84 (17.9282, -43.384) -> (21.6698, -47.1257) centre (21.9203, -43.1335) ccw construction
  line L61 (21.6698, -47.1257) -> (26.2105, -51.6664) construction
  line L62 (29.746, -55.2019) -> (42.4264, -67.8823) construction
  line L63 (42.4264, -67.8823) -> (37.1244, -73.1843) construction
  arc A85 (34.1909, -73.0707) -> (37.1244, -73.1843) centre (35.7102, -71.7701) ccw construction
  line L64 (34.1909, -73.0707) -> (25.4187, -62.8242) construction
  arc A86 (24.842, -61.8893) -> (25.4187, -62.8242) centre (28.1154, -60.5155) ccw construction
  line L65 (24.842, -61.8893) -> (24.3148, -60.6331) construction
  line L66 (24.3148, -60.6331) -> (29.746, -55.2019) construction
  arc A87 (-90.4395, 37.7453) -> (-97.9653, 2.6059) centre (0, 0) ccw construction
  arc A88 (-87.1795, 38.3892) -> (-90.4395, 37.7453) centre (-88.5938, 36.975) ccw construction
  line L67 (-87.1795, 38.3892) -> (-83.085, 34.2947) construction
  arc A89 (-83.085, 34.2947) -> (-76.014, 34.2947) centre (-79.5495, 37.8302) ccw construction
  line L68 (-76.014, 34.2947) -> (-67.8823, 42.4264) construction
  line L69 (-67.8823, 42.4264) -> (-47.1257, 21.6698) construction
  arc A90 (-47.1257, 21.6698) -> (-43.384, 17.9282) centre (-43.1335, 21.9203) ccw construction
  line L70 (-43.384, 17.9282) -> (-26.8701, 1.4142) construction
  arc A91 (-26.8701, -1.4142) -> (-26.8701, 1.4142) centre (-28.2843, 0) ccw construction
  line L71 (-26.8701, -1.4142) -> (-43.384, -17.9282) construction
  arc A92 (-43.384, -17.9282) -> (-47.1257, -21.6698) centre (-43.1335, -21.9203) ccw construction
  line L72 (-47.1257, -21.6698) -> (-67.8823, -42.4264) construction
  line L73 (-67.8823, -42.4264) -> (-76.014, -34.2947) construction
  arc A93 (-76.014, -34.2947) -> (-83.085, -34.2947) centre (-79.5495, -37.8302) ccw construction
  line L74 (-83.085, -34.2947) -> (-87.1795, -38.3892) construction
  arc A94 (-90.4395, -37.7453) -> (-87.1795, -38.3892) centre (-88.5938, -36.975) ccw construction
  arc A95 (-97.9653, -2.6059) -> (-90.4395, -37.7453) centre (0, 0) ccw construction
  arc A96 (-97.9653, -2.6059) -> (-97.9653, 2.6059) centre (-101, 0) ccw construction
  arc A97 (-93.0503, 48.6481) -> (-93.0503, -48.6481) centre (0, 0) ccw construction
  arc A98 (-93.0503, -48.6481) -> (-88.2704, -49.3795) centre (-90.3917, -47.2582) ccw construction
  line L75 (-88.2704, -49.3795) -> (-85.2064, -46.3155) construction
  arc A99 (-73.8927, -46.3155) -> (-85.2064, -46.3155) centre (-79.5495, -51.9723) ccw construction
  line L76 (-73.8927, -46.3155) -> (-46.3155, -73.8927) construction
  arc A100 (-46.3155, -85.2064) -> (-46.3155, -73.8927) centre (-51.9723, -79.5495) ccw construction
  line L77 (-46.3155, -85.2064) -> (-49.3795, -88.2704) construction
  arc A101 (-49.3795, -88.2704) -> (-48.6481, -93.0503) centre (-47.2582, -90.3917) ccw construction
  arc A102 (-48.6481, -93.0503) -> (-45.42, -94.668) centre (0, 0) ccw construction
  arc A103 (-45.42, -94.668) -> (-43.0355, -94.1655) centre (-44.5548, -92.8648) ccw construction
  line L78 (-43.0355, -94.1655) -> (-18.3802, -65.3664) construction
  arc A104 (-17.477, -64.7643) -> (-18.3802, -65.3664) centre (-16.8609, -66.6671) ccw construction
  line L79 (-17.477, -64.7643) -> (-0.6161, -59.3045) construction
  arc A105 (0.6161, -59.3045) -> (-0.6161, -59.3045) centre (0, -61.2072) ccw construction
  line L80 (0.6161, -59.3045) -> (17.477, -64.7643) construction
  arc A106 (18.3802, -65.3664) -> (17.477, -64.7643) centre (16.8609, -66.6671) ccw construction
  line L81 (18.3802, -65.3664) -> (43.0355, -94.1655) construction
  arc A107 (43.0355, -94.1655) -> (45.42, -94.668) centre (44.5548, -92.8648) ccw construction
  arc A108 (45.42, -94.668) -> (48.6481, -93.0503) centre (0, 0) ccw construction
  arc A109 (48.6481, -93.0503) -> (49.3795, -88.2704) centre (47.2582, -90.3917) ccw construction
  line L82 (49.3795, -88.2704) -> (46.3155, -85.2064) construction
  arc A110 (46.3155, -73.8927) -> (46.3155, -85.2064) centre (51.9723, -79.5495) ccw construction
  line L83 (46.3155, -73.8927) -> (73.8927, -46.3155) construction
  arc A111 (85.2064, -46.3155) -> (73.8927, -46.3155) centre (79.5495, -51.9723) ccw construction
  line L84 (85.2064, -46.3155) -> (88.2704, -49.3795) construction
  arc A112 (88.2704, -49.3795) -> (93.0503, -48.6481) centre (90.3917, -47.2582) ccw construction
  arc A113 (93.0503, -48.6481) -> (93.0503, 48.6481) centre (0, 0) ccw construction
  arc A114 (93.0503, 48.6481) -> (88.2704, 49.3795) centre (90.3917, 47.2582) ccw construction
  line L85 (88.2704, 49.3795) -> (85.2064, 46.3155) construction
  arc A115 (73.8927, 46.3155) -> (85.2064, 46.3155) centre (79.5495, 51.9723) ccw construction
  line L86 (73.8927, 46.3155) -> (46.3155, 73.8927) construction
  arc A116 (46.3155, 85.2064) -> (46.3155, 73.8927) centre (51.9723, 79.5495) ccw construction
  line L87 (46.3155, 85.2064) -> (49.3795, 88.2704) construction
  arc A117 (49.3795, 88.2704) -> (48.6481, 93.0503) centre (47.2582, 90.3917) ccw construction
  arc A118 (48.6481, 93.0503) -> (11.8382, 104.3305) centre (0, 0) ccw construction
  arc A119 (11.8382, 104.3305) -> (8.5, 101.3496) centre (11.5, 101.3496) ccw construction
  line L88 (8.5, 101.3496) -> (8.5, 90.5) construction
  arc A120 (7, 89) -> (8.5, 90.5) centre (7, 90.5) ccw construction
  line L89 (7, 89) -> (-7, 89) construction
  arc A121 (-8.5, 90.5) -> (-7, 89) centre (-7, 90.5) ccw construction
  line L90 (-8.5, 90.5) -> (-8.5, 101.3496) construction
  arc A122 (-8.5, 101.3496) -> (-11.8382, 104.3305) centre (-11.5, 101.3496) ccw construction
  arc A123 (-11.8382, 104.3305) -> (-48.6481, 93.0503) centre (0, 0) ccw construction
  arc A124 (-48.6481, 93.0503) -> (-49.3795, 88.2704) centre (-47.2582, 90.3917) ccw construction
  line L91 (-49.3795, 88.2704) -> (-46.3155, 85.2064) construction
  arc A125 (-46.3155, 73.8927) -> (-46.3155, 85.2064) centre (-51.9723, 79.5495) ccw construction
  line L92 (-46.3155, 73.8927) -> (-73.8927, 46.3155) construction
  arc A126 (-85.2064, 46.3155) -> (-73.8927, 46.3155) centre (-79.5495, 51.9723) ccw construction
  line L93 (-85.2064, 46.3155) -> (-88.2704, 49.3795) construction
  arc A127 (-88.2704, 49.3795) -> (-93.0503, 48.6481) centre (-90.3917, 47.2582) ccw construction
  circle A128 centre (0, 0) radius 101 construction
  circle A129 centre (-90.3659, -45.1111) radius 1.6
  line L94 (-41.3657, -27.2236) -> (-27.2236, -41.3657) construction
  line L95 (-34.2947, -34.2947) -> (-55.1543, -55.1543) construction
  line L96 (-46.669, -63.6396) -> (-63.6396, -46.669) construction
  circle A130 centre (-45.1111, -90.3659) radius 1.6
  line L97 (-22, 0) -> (-101, 0) construction